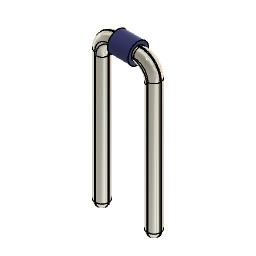
Adjustable_Jumper (Autodesk Fusion 360 design; units mm, degrees)
Autodesk Fusion 360 part; units mm, degrees
sketch "Sketch1" plane through (0, 0, 0) normal (1, 0, 0) x (0, 1, 0)
  circle A0 centre (0, 0) radius 0.5
  line L0 (0.325, -0.325) -> (-0.325, -0.325)
  line L1 (-0.325, -0.325) -> (-0.325, 0.325)
  line L2 (-0.325, 0.325) -> (0.325, 0.325)
  line L3 (0.325, 0.325) -> (0.325, -0.325)
  line L4 (0.325, -0.325) -> (-0.325, 0.325) construction
  line L5 (-0.325, -0.325) -> (0.325, 0.325) construction
  dimension "d1" = 1
  dimension "d2" = 0.65
  dimension "d3" = 0.65
  constraint coincident A0.centre origin
  constraint horizontal L0
  constraint perpendicular L0 L1
  constraint parallel L0 L2
  constraint parallel L1 L3
  constraint coincident L4 A0.centre
  constraint coincident L5 A0.centre
  measures "d1" diameter of A0
  measures "d2" distance of L1.end L2.end
  measures "d3" distance of L0.end L1.end
extrude "Extrude1" add sketch "Sketch1" along normal blind 1 contours A0 | L0 L1 L2 L3
sketch "Sketch2" plane through (1, 0, 0) normal (1, 0, 0) x (0, 1, 0)
  circle A0 centre (0, 0) radius 0.5
  line L0 (0.325, -0.325) -> (-0.325, -0.325)
  line L1 (-0.325, -0.325) -> (-0.325, 0.325)
  line L2 (-0.325, 0.325) -> (0.325, 0.325)
  line L3 (0.325, 0.325) -> (0.325, -0.325)
  line L4 (0.325, -0.325) -> (-0.325, 0.325) construction
  line L5 (-0.325, -0.325) -> (0.325, 0.325) construction
  dimension "d8" = 0.65
  dimension "d9" = 0.65
  constraint horizontal L0
  constraint perpendicular L0 L1
  constraint parallel L0 L2
  constraint parallel L1 L3
  constraint coincident L4 A0.centre
  constraint coincident L5 A0.centre
  constraint coincident A0.centre origin
  measures "d8" distance of L1.end L2.end
  measures "d9" distance of L0.end L1.end
extrude "Extrude2" add sketch "Sketch2" along normal blind 1.095 contours L0 L1 L2 L3
extrude "Extrude3" add sketch "Sketch1" against normal blind 1.095 contours L0 L1 L2 L3
sketch "Sketch3" plane through (0, 0, -0.325) normal (0, 0, -1) x (1, 0, 0)
  line L0 (1, 0.325) -> (1, -0.325)
  line L1 (1, -0.325) -> (2.095, -0.325)
  line L2 (2.095, -0.325) -> (2.095, 0.325)
  line L3 (2.095, 0.325) -> (1, 0.325)
  line L4 (2.095, 0.325) -> (1.445, 0.325)
  line L5 (1.445, 0.325) -> (1.445, -0.325)
  line L6 (1.445, -0.325) -> (2.095, -0.325)
  line L7 (2.095, -0.325) -> (2.095, 0.325)
  line L8 (2.095, 0.325) -> (1.445, -0.325) construction
  line L9 (1.445, 0.325) -> (2.095, -0.325) construction
  point P0 (1.77, 0)
  dimension "d14" = 0.65
  dimension "d15" = 0.65
  constraint horizontal L4
  constraint perpendicular L4 L5
  constraint parallel L4 L6
  constraint parallel L5 L7
  constraint coincident L8 P0
  constraint coincident L9 P0
  constraint coincident L3 L2.end
  constraint coincident L2.end L7
  measures "d14" distance of L5 L7
  measures "d15" distance of L4 L6
sketch "Sketch4" plane through (0, 0, -0.325) normal (0, 0, -1) x (1, 0, 0)
  line L0 (0, -0.325) -> (0, 0.325)
  line L1 (0, 0.325) -> (-1.095, 0.325)
  line L2 (-1.095, 0.325) -> (-1.095, -0.325)
  line L3 (-1.095, -0.325) -> (0, -0.325)
  line L4 (-0.445, -0.325) -> (-1.095, -0.325)
  line L5 (-1.095, -0.325) -> (-1.095, 0.325)
  line L6 (-1.095, 0.325) -> (-0.445, 0.325)
  line L7 (-0.445, 0.325) -> (-0.445, -0.325)
  line L8 (-0.445, -0.325) -> (-1.095, 0.325) construction
  line L9 (-1.095, -0.325) -> (-0.445, 0.325) construction
  point P0 (-0.77, 0)
  dimension "d17" = 0.65
  dimension "d18" = 0.65
  constraint horizontal L4
  constraint perpendicular L4 L5
  constraint parallel L4 L6
  constraint parallel L5 L7
  constraint coincident L8 P0
  constraint coincident L9 P0
  constraint coincident L3 L4.start
  constraint coincident L1.end L5
  measures "d17" distance of L5 L7
  measures "d18" distance of L4 L6
extrude "Extrude4" add sketch "Sketch4" sketch "Sketch3" along normal blind 7 contours L1 L2 L3 L4 L5 L6 L7 of sketch 2 contours L1 L2 L3 L4 L5 L6 L7
fillet "Fillet1" radius 0.5 2 edges at (-0.445, 0, -0.325) (1.445, 0, -0.325)
fillet "Fillet2" radius 1 2 edges at (-1.095, 0, 0.325) (2.095, 0, 0.325)
fillet "Fillet3" radius 0.3 28 edges at (-0.77, -0.325, -7.325) (-0.445, 0, -7.325) (-0.77, 0.325, -7.325) (-1.095, 0, -7.325) (-0.3175, -0.325, -0.4884) (-0.445, -0.325, -4.0735) (-0.0475, -0.325, 0.325) (-0.8021, -0.325, 0.0321) (-1.095, -0.325, -4) (-0.0475, 0.325, 0.325) (-0.8021, 0.325, 0.0321) (-1.095, 0.325, -4) (-0.3175, 0.325, -0.4884) (-0.445, 0.325, -4.0735) (1.0475, -0.325, 0.325) (1.8021, -0.325, 0.0321) (2.095, -0.325, -4) (1.445, -0.325, -4.0735) (1.3175, -0.325, -0.4884) (2.095, 0.325, -4) (1.8021, 0.325, 0.0321) (1.0475, 0.325, 0.325) (1.3175, 0.325, -0.4884) (1.445, 0.325, -4.0735) (1.77, 0.325, -7.325) (2.095, 0, -7.325) (1.77, -0.325, -7.325) (1.445, 0, -7.325)
equation "d1 = jumperWidth"
equation "d2 = d3"
equation "d3 = d1 * 0.65"
equation "jumperWidth = 1 mm"
equation "jumperBaseLenght = 1 mm"
equation "d6 = jumperBaseLenght"
equation "d8 = jumperWidth * 0.65"
equation "d9 = d8"
equation "d10 = ( ( 2.54 * ceil(( jumperBaseLenght + 1.3 * jumperWidth ) / 2.54 mm) ) * 1 mm + 0.65 * jumperWidth - jumperBaseLenght ) / 2"
equation "d12 = -( ( 2.54 * ceil(( jumperBaseLenght + 1.3 * jumperWidth ) / 2.54 mm) ) * 1 mm + 0.65 * jumperWidth - jumperBaseLenght ) / 2"
equation "d14 = jumperWidth * 0.65"
equation "d15 = d14"
equation "d17 = jumperWidth * 0.65"
equation "d18 = d17"
equation "d26 = 0.3 * jumperWidth"
